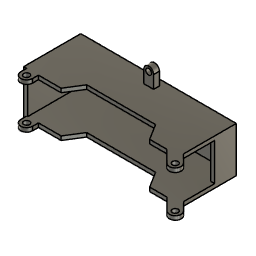
電池ボックス v6 (Autodesk Fusion 360 design; units mm, degrees)
Autodesk Fusion 360 part; units mm, degrees
sketch "スケッチ1" plane through (0, 0, 0) normal (1, 0, 0) x (0, 1, 0)
  line L0 (0, 0) -> (31, 0)
  line L1 (31, 0) -> (31, 25)
  line L2 (31, 25) -> (0, 25)
  line L3 (0, 25) -> (0, 0)
  line L4 (0, 0) -> (0, 12.5)
  line L5 (0, 12.5) -> (0, 2)
  line L6 (0, 12.5) -> (0, 23)
  line L7 (15.5, 0) -> (0, 0)
  line L8 (15.5, 2) -> (2, 2)
  line L9 (15.5, 2) -> (29, 2)
  line L10 (2, 2) -> (2, 23)
  line L11 (29, 2) -> (29, 23)
  line L12 (2, 23) -> (29, 23)
  dimension "d1" = 31
  dimension "d2" = 12.5
  dimension "d3" = 10.5
  dimension "d4" = 10.5
  dimension "d5" = 2
  dimension "d6" = 13.5
  dimension "d7" = 13.5
  dimension "d8" = 21
  dimension "d9" = 21
  constraint horizontal L0
  constraint vertical L1
  constraint horizontal L2
  constraint vertical L3
  constraint coincident L0.start L3.end
  constraint perpendicular L0 L4
  constraint parallel L3 L5
  constraint parallel L3 L6
  constraint midpoint L0 L7.start
  constraint perpendicular L1 L9
  constraint perpendicular L8 L10
  constraint perpendicular L9 L11
  measures "d1" distance of L0.start L0.end
  measures "d2" distance of L0.start L4.end
  measures "d3" distance of L4.end L5.end
  measures "d4" distance of L4.end L6.end
  measures "d5" distance of L7.start L8.start
  measures "d6" distance of L8.start L8.end
  measures "d7" distance of L8.start L9.end
  measures "d8" distance of L8.end L10.end
  measures "d9" distance of L9.end L11.end
extrude "押し出し1" add sketch "スケッチ1" along normal blind 75 makes body 1
sketch "スケッチ2" plane through (0, 31, 0) normal (0, 1, 0) x (-1, 0, 0)
sketch "スケッチ3" plane through (0, 0, 0) normal (1, 0, 0) x (0, 1, 0)
sketch "スケッチ4" plane through (0, 0, 0) normal (0, 1, 0) x (1, 0, 0)
sketch "スケッチ5" plane through (0, 0, 0) normal (1, 0, 0) x (0, 1, 0)
  line L0 (0, 0) -> (2, 0)
  line L1 (2, 0) -> (2, 25)
  line L2 (2, 25) -> (0, 25)
  line L3 (0, 25) -> (0, 0)
  constraint horizontal L0
  constraint vertical L1
  constraint horizontal L2
  constraint vertical L3
  constraint coincident L0.start L3.end
extrude "押し出し2" cut sketch "スケッチ5" along normal blind 75 bodies 1
sketch "スケッチ6" plane through (0, 0, 0) normal (0, 0, 1) x (1, 0, 0)
  circle A0 centre (77, 0) radius 1
  arc A1 (75.5858, -1.4142) -> (78.3586, 1.4677) centre (77, 0) ccw
  line L0 (78.3586, 1.4677) -> (75, 4)
  line L1 (75, 4) -> (75, 2)
  line L2 (75, 2) -> (73, 2)
  line L3 (73, 2) -> (75.5858, -1.4142)
  dimension "d17" = 2
  constraint coincident A0.centre A1.centre
  constraint vertical L1
  constraint perpendicular L1 L2
  measures "d17" radius of A1
extrude "押し出し3" add sketch "スケッチ6" along normal blind 2 bodies 1
sketch "スケッチ7" plane through (0, 0, 25) normal (0, 0, 1) x (-1, 0, 0)
  line L0 (0, -2) -> (-75, -2)
  line L1 (-75, -2) -> (-75, -31)
  line L2 (-75, -31) -> (0, -31)
  line L3 (0, -31) -> (0, -2)
  circle A0 centre (-77, 0) radius 1
  arc A1 (-75.5967, 1.425) -> (-78.4142, -1.4142) centre (-77, 0) ccw
  line L4 (-75.5967, 1.425) -> (-73, -2)
  line L5 (-75, -2) -> (-75, -4)
  line L6 (-78.4142, -1.4142) -> (-75, -4)
  line L7 (-75, -2) -> (-73, -2)
  dimension "d20" = 2
  constraint coincident A0.centre A1.centre
  constraint coincident L0 L4.end
  constraint coincident L0.end L1.start
  constraint coincident L1 L5.end
  constraint perpendicular L0 L5
  measures "d20" radius of A1
extrude "押し出し4" add sketch "スケッチ7" against normal blind 2 contours L0 L1 A1 L4 L5 L6 L7 bodies 1
sketch "スケッチ8" plane through (0, 0, 0) normal (0, 0, 1) x (1, 0, 0)
sketch "スケッチ9" plane through (0, 0, 0) normal (1, 0, 0) x (0, 1, 0)
sketch "スケッチ10" plane through (0, 0, 0) normal (0, 1, 0) x (1, 0, 0)
sketch "スケッチ11" plane through (0, 0, 0) normal (1, 0, 0) x (0, 1, 0)
  line L0 (31, 25) -> (9, 25)
  line L1 (9, 25) -> (9, 0)
  line L2 (9, 0) -> (31, 0)
  line L3 (31, 0) -> (31, 25)
  constraint horizontal L0
  constraint vertical L1
  constraint horizontal L2
  constraint vertical L3
extrude "押し出し5" add sketch "スケッチ11" against normal blind 2 bodies 1
sketch "スケッチ12" plane through (0, 0, 0) normal (1, 0, 0) x (0, 1, 0)
  line L0 (29, 23) -> (17, 23)
  line L1 (2, 23) -> (17, 23)
  line L2 (17, 23) -> (17, 2)
  line L3 (17, 2) -> (2, 2)
  line L4 (2, 2) -> (2, 23)
  constraint horizontal L0
  constraint horizontal L1
  constraint vertical L2
  constraint horizontal L3
  constraint vertical L4
extrude "押し出し6" add sketch "スケッチ12" along normal blind 75 bodies 1
sketch "スケッチ13" plane through (0, 0, 0) normal (1, 0, 0) x (0, 1, 0)
  line L0 (2, 23) -> (17, 23)
  line L1 (17, 23) -> (17, 2)
  line L2 (17, 2) -> (2, 2)
  line L3 (2, 2) -> (2, 23)
  constraint horizontal L0
  constraint vertical L1
  constraint horizontal L2
  constraint vertical L3
extrude "押し出し7" cut sketch "スケッチ13" along normal blind 73 bodies 1
sketch "スケッチ14" plane through (0, 0, 25) normal (0, 0, 1) x (-1, 0, 0)
  circle A0 centre (-77, 0) radius 1
  line L0 (0, -2) -> (-73, -2)
  line L1 (-73, -2) -> (-75.5967, 1.425)
  arc A1 (-75.5967, 1.425) -> (-78.4142, -1.4142) centre (-77, 0) ccw
  line L2 (-78.4142, -1.4142) -> (-75, -4)
  line L3 (-75, -4) -> (-75, -31)
  line L4 (-75, -31) -> (2, -31)
  line L5 (2, -31) -> (2, -9)
  line L6 (2, -9) -> (0, -9)
  line L7 (0, -9) -> (0, -2)
  line L8 (0, -2) -> (-3, -2)
  line L9 (0, -2) -> (0, 1.5)
  line L10 (-3, -2) -> (-3, 1.5)
  circle A2 centre (-1.5, 1.5) radius 1
  arc A3 (0, 1.5) -> (-3, 1.5) centre (-1.5, 1.5) ccw
  constraint coincident L0.start L7.end
  constraint coincident L0 L8.end
  constraint perpendicular L7 L8
  constraint perpendicular L0 L9
  constraint perpendicular L8 L10
  constraint coincident A2.centre A3.centre
extrude "押し出し8" add sketch "スケッチ14" against normal blind 25 contours L0 L8 L9 L10 A3 bodies 1
sketch "スケッチ15" plane through (0, 0, 25) normal (0, 0, 1) x (-1, 0, 0)
  circle A0 centre (-1.5, 1.5) radius 1
  circle A1 centre (-77, 0) radius 1
  line L0 (-3, -2) -> (-73, -2)
  line L1 (-73, -2) -> (-75.5967, 1.425)
  arc A2 (-75.5967, 1.425) -> (-78.4142, -1.4142) centre (-77, 0) ccw
  line L2 (-78.4142, -1.4142) -> (-75, -4)
  line L3 (-75, -4) -> (-75, -31)
  line L4 (-75, -31) -> (2, -31)
  line L5 (2, -31) -> (2, -9)
  line L6 (2, -9) -> (0, -9)
  line L7 (0, -9) -> (0, 1.5)
  arc A3 (0, 1.5) -> (-3, 1.5) centre (-1.5, 1.5) ccw
  line L8 (-3, 1.5) -> (-3, -2)
  line L9 (-3, 1.5) -> (-3, -2)
  line L10 (0, -2) -> (-3, -2)
  line L11 (0, -2) -> (0, 1.5)
  arc A4 (0, 1.5) -> (-3, 1.5) centre (-1.5, 1.5) ccw
  circle A5 centre (-1.5, 1.5) radius 1
  constraint coincident A3.end L8.start
  constraint coincident L0.start L8.end
  constraint coincident L7 L10.start
  constraint perpendicular L8 L10
  constraint coincident L7.end A3.start
  constraint coincident A0.centre A3.centre
  constraint concentric A4 A5
extrude "押し出し9" cut sketch "スケッチ15" against normal blind 23 contours L7 A3 L8 L9 L10 L11 A4 bodies 1
sketch "スケッチ16" plane through (0, 0, 25) normal (0, 0, 1) x (-1, 0, 0)
  line L0 (0, -2) -> (-73, -2)
  line L1 (-73, -2) -> (-75.5967, 1.425)
  arc A0 (-75.5967, 1.425) -> (-78.4142, -1.4142) centre (-77, 0) ccw
  line L2 (-78.4142, -1.4142) -> (-75, -4)
  line L3 (-75, -4) -> (-75, -31)
  line L4 (-75, -31) -> (2, -31)
  line L5 (2, -31) -> (2, -9)
  line L6 (2, -9) -> (0, -9)
  line L7 (0, -9) -> (0, -2)
  circle A1 centre (-77, 0) radius 1
  line L8 (-3, 1.5) -> (-3, -2)
  line L9 (-3, -2) -> (0, -2)
  line L10 (0, 1.5) -> (0, -2)
  arc A2 (0, 1.5) -> (-3, 1.5) centre (-1.5, 1.5) ccw
  circle A3 centre (-1.5, 1.5) radius 1
  constraint coincident L0 L8.end
  constraint perpendicular L0 L8
  constraint coincident L0.start L7.end
  constraint perpendicular L0 L10
  constraint concentric A2 A3
extrude "押し出し10" add sketch "スケッチ16" against normal blind 2 contours L0 L8 L9 L10 A2 bodies 1
sketch "スケッチ17" plane through (0, 0, 25) normal (0, 0, 1) x (-1, 0, 0)
  circle A0 centre (-1.5, 1.5) radius 1
  line L0 (-3, -2) -> (-73, -2)
  line L1 (-73, -2) -> (-75.5967, 1.425)
  arc A1 (-75.5967, 1.425) -> (-78.4142, -1.4142) centre (-77, 0) ccw
  line L2 (-78.4142, -1.4142) -> (-75, -4)
  line L3 (-75, -4) -> (-75, -31)
  line L4 (-75, -31) -> (2, -31)
  line L5 (2, -31) -> (2, -9)
  line L6 (2, -9) -> (0, -9)
  line L7 (0, -9) -> (0, 1.5)
  arc A2 (0, 1.5) -> (-3, 1.5) centre (-1.5, 1.5) ccw
  line L8 (-3, 1.5) -> (-3, -2)
  circle A3 centre (-77, 0) radius 1
  circle A4 centre (4, 1) radius 0.95
  dimension "d35" = 1.9
  measures "d35" diameter of A4
sketch "スケッチ18" plane through (0, 0, 0) normal (0, 0, 1) x (1, 0, 0)
  circle A0 centre (-6.5, -1) radius 0.95
  dimension "d38" = 1.9
  measures "d38" diameter of A0
sketch "スケッチ19" plane through (0, 31, 0) normal (0, 1, 0) x (-1, 0, 0)
sketch "スケッチ20" plane through (0, 0, 0) normal (0, 0, 1) x (1, 0, 0)
  line L0 (15, 2) -> (20, 10)
  line L1 (20, 10) -> (55, 10)
  line L2 (55, 10) -> (60, 2)
  line L3 (15, 2) -> (60, 2)
  constraint horizontal L1
  constraint horizontal L3
extrude "押し出し13" cut sketch "スケッチ20" along normal blind 2 bodies 1
sketch "スケッチ21" plane through (0, 0, 25) normal (0, 0, 1) x (-1, 0, 0)
  circle A0 centre (-1.5, 1.5) radius 1
  line L0 (-3, -2) -> (-73, -2)
  line L1 (-73, -2) -> (-75.5967, 1.425)
  arc A1 (-75.5967, 1.425) -> (-78.4142, -1.4142) centre (-77, 0) ccw
  line L2 (-78.4142, -1.4142) -> (-75, -4)
  line L3 (-75, -4) -> (-75, -31)
  line L4 (-75, -31) -> (2, -31)
  line L5 (2, -31) -> (2, -9)
  line L6 (2, -9) -> (0, -9)
  line L7 (0, -9) -> (0, 1.5)
  arc A2 (0, 1.5) -> (-3, 1.5) centre (-1.5, 1.5) ccw
  line L8 (-3, 1.5) -> (-3, -2)
  circle A3 centre (-77, 0) radius 1
  line L9 (-15, -2) -> (-20, -10)
  line L10 (-60, -2) -> (-55, -10)
  line L11 (-55, -10) -> (-20, -10)
  constraint coincident L0 L9.start
  constraint coincident L0 L10.start
  constraint parallel L0 L11
extrude "押し出し14" cut sketch "スケッチ21" against normal blind 2 contours L0 L9 L10 L11 bodies 1
sketch "スケッチ22" plane through (0, 0, 0) normal (0, 0, 1) x (1, 0, 0)
sketch "スケッチ23" plane through (0, 31, 0) normal (0, 1, 0) x (-1, 0, 0)
sketch "スケッチ24" plane through (0, 0, 0) normal (0, 0, 1) x (1, 0, 0)
sketch "スケッチ25" plane through (0, 0, 0) normal (0, 1, 0) x (1, 0, 0)
  line L0 (75, 0) -> (36.5, 0)
  line L1 (36.5, 0) -> (36.5, -25)
  line L2 (36.5, 0) -> (34, 0)
  line L3 (36.5, 0) -> (39, 0)
  line L4 (39, 0) -> (34, 0)
  line L5 (34, 0) -> (34, 8)
  line L6 (34, 8) -> (39, 8)
  line L7 (39, 8) -> (39, 0)
  line L8 (34, 8) -> (34, 5.5)
  line L9 (34, 5.5) -> (36.5, 5.5)
  circle A0 centre (36.5, 5.5) radius 1.5
  arc A1 (39, 5.4984) -> (34, 5.5) centre (36.5, 5.5) ccw
  dimension "d46" = 38.5
  dimension "d47" = 2.5
  dimension "d48" = 2.5
  dimension "d49" = 2.5
  dimension "d50" = 2.5
  dimension "d51" = 3
  constraint horizontal L0
  constraint perpendicular L0 L1
  constraint perpendicular L1 L2
  constraint perpendicular L1 L3
  constraint horizontal L4
  constraint vertical L5
  constraint horizontal L6
  constraint vertical L7
  constraint perpendicular L6 L8
  constraint perpendicular L7 L9
  constraint coincident L9.end A0.centre
  constraint coincident L7 A1.start
  measures "d46" distance of L0.start L0.end
  measures "d47" distance of L0.end L2.end
  measures "d48" distance of L0.end L3.end
  measures "d49" distance of L5.end L8.end
  measures "d50" distance of L8.end L9.end
  measures "d51" diameter of A0
extrude "押し出し15" add sketch "スケッチ25" along normal blind 15 contours L0 L2 L3 L4 L5 L7 A1 bodies 1
extrude "押し出し16" cut 1 faces at (36.4626, 0, -1.3347) along direction (0, 1, 0) blind 13 on bodies 1 bodies 1
sketch "スケッチ26" plane through (0, 0, 0) normal (0, 1, 0) x (1, 0, 0)
  line L0 (-2, -25) -> (36.5, -25)
  line L1 (36.5, -25) -> (36.5, -30.5)
  circle A0 centre (36.5, -30.5) radius 1.5
  arc A1 (34, -30.5) -> (39, -30.5) centre (36.5, -30.5) ccw
  line L2 (34, -30.5) -> (34, -25)
  line L3 (39.2947, -30.5) -> (39.2947, -25)
  line L4 (39.2947, -25) -> (34, -25)
  line L5 (39, -30.5) -> (39, -25)
  dimension "d56" = 38.5
  dimension "d57" = 5.5
  dimension "d58" = 3
  dimension "d59" = 2.5
  constraint horizontal L0
  constraint perpendicular L0 L1
  constraint coincident L1.end A0.centre
  constraint coincident L0 L2.end
  constraint tangent A1 L2
  constraint perpendicular L0 L2
  constraint parallel L2 L3
  constraint perpendicular L2 L4
  constraint coincident L4 L5.end
  constraint tangent A1 L5
  constraint perpendicular L4 L5
  measures "d56" distance of L0.start L0.end
  measures "d57" distance of L0.end L1.end
  measures "d58" diameter of A0
  measures "d59" radius of A1
extrude "押し出し17" add sketch "スケッチ26" along normal blind 15 bodies 1
extrude "押し出し18" cut 1 faces at (36.5374, 0, 26.3347) along direction (0, 1, 0) blind 20 on bodies 1 bodies 1
sketch "スケッチ27" plane through (0, 0, 0) normal (0, 1, 0) x (1, 0, 0)
sketch "スケッチ28" plane through (0, 0, 0) normal (0, 1, 0) x (1, 0, 0)
  line L0 (-2, -2) -> (-2, -21)
  line L1 (-2, -21) -> (75, -21)
  line L2 (75, -23) -> (75, -21)
  line L3 (75, -23) -> (-2, -23)
  line L4 (-2, -23) -> (-2, -21)
  constraint vertical L0
  constraint perpendicular L0 L1
  constraint perpendicular L1 L2
  constraint perpendicular L2 L3
  constraint perpendicular L1 L4
extrude "押し出し19" cut sketch "スケッチ28" along normal blind 70 bodies 1 makes body 2 at (38, 25.6667, 0)
move_body "移動4" bodies 1 to x (1, 0, 0) y (0, 1, 0) z (0, 0, 1) at (0, 0, -2)
sketch "スケッチ29" plane through (0, 0, 0) normal (0, 1, 0) x (1, 0, 0)
sketch "スケッチ30" plane through (0, 13, 0) normal (0, -1, 0) x (1, 0, 0)
extrude "押し出し20" cut 1 faces at (36.4626, 15, -1.3347) along direction (0, -1, 0) blind 40 on bodies 2 bodies 2
sketch "スケッチ31" plane through (0, 0, 0) normal (0, 1, 0) x (1, 0, 0)
  line L0 (39, 0) -> (39, 4)
  line L1 (39, 0) -> (34, 0)
  line L2 (34, 0) -> (34, 4)
  circle A0 centre (36.5, 6.5) radius 1.5
  arc A1 (39, 6.5) -> (34, 6.5) centre (36.5, 6.5) ccw
  line L3 (34, 6.5) -> (34, 4)
  line L4 (39, 6.5) -> (39, 4)
  constraint vertical L0
  constraint perpendicular L0 L1
  constraint perpendicular L1 L2
  constraint coincident A0.centre A1.centre
  constraint parallel L2 L3
extrude "押し出し21" add sketch "スケッチ31" along normal blind 14 bodies 2
extrude "押し出し22" cut 1 faces at (36.5374, 0, -1.6681) along direction (0, 1, 0) blind 12 on bodies 2 bodies 2
sketch "スケッチ32" plane through (0, 29, 0) normal (0, -1, 0) x (1, 0, 0)
  line L0 (75, 21) -> (0, 21)
  line L1 (0, 21) -> (0, 2)
  line L2 (0, 2) -> (75, 2)
  line L3 (75, 2) -> (75, 21)
  line L4 (39, 23) -> (39, 27)
  line L5 (34, 23) -> (34, 27)
  line L6 (34, 23) -> (39, 23)
  circle A0 centre (36.5, 29.5) radius 1.5
  arc A1 (39, 29.5) -> (34, 29.5) centre (36.5, 29.5) ccw
  line L7 (39, 29.5) -> (39, 27)
  line L8 (34, 29.5) -> (34, 27)
  dimension "d78" = 3
  constraint perpendicular L0 L4
  constraint vertical L5
  constraint perpendicular L4 L6
  constraint coincident A0.centre A1.centre
  constraint parallel L4 L7
  constraint parallel L5 L8
  measures "d78" diameter of A0
extrude "押し出し23" add sketch "スケッチ32" along normal blind 17 contours L4 L5 L6 A1 L7 L8 bodies 1
extrude "押し出し24" cut 1 faces at (36.5374, 29, 24.6681) along direction (0, -1, 0) blind 15 on bodies 1 bodies 1
sketch "スケッチ33" plane through (0, 0, 0) normal (0, 1, 0) x (1, 0, 0)
sketch "スケッチ34" plane through (0, 0, 0) normal (0, 1, 0) x (1, 0, 0)
sketch "スケッチ35" plane through (0, 0, 0) normal (0, 1, 0) x (1, 0, 0)
sketch "スケッチ36" plane through (0, 0, 23) normal (0, 0, 1) x (-1, 0, 0)
sketch "スケッチ37" plane through (0, 0, 0) normal (1, 0, 0) x (0, 1, 0)
sketch "スケッチ38" plane through (0, 0, 2) normal (0, 0, 1) x (-1, 0, 0)
sketch "スケッチ39" plane through (0, 0, 0) normal (0, 1, 0) x (1, 0, 0)
move_body "移動5" bodies 2 1 to x (1, 0, 0) y (0, 1, 0) z (0, 0, 1) at (2, 0, 0)
sketch "スケッチ40" plane through (0, 0, 0) normal (1, 0, 0) x (0, 1, 0)
  line L0 (9, 23) -> (31, 23)
  line L1 (31, 23) -> (31, 0)
  line L2 (31, 0) -> (9, 0)
  line L3 (9, 0) -> (9, 23)
  constraint horizontal L0
  constraint vertical L1
  constraint horizontal L2
  constraint vertical L3
extrude "押し出し25" cut sketch "スケッチ40" along normal blind 2 bodies 1 2
sketch "スケッチ41" plane through (0, 0, 0) normal (0, 0, 1) x (1, 0, 0)
  line L0 (5, 2) -> (0.471, 2)
  line L1 (0.471, 2) -> (0.471, -4.3481)
  line L2 (0.471, -4.3481) -> (5, -4.3481)
  line L3 (5, -4.3481) -> (5, 2)
  constraint horizontal L0
  constraint vertical L1
  constraint horizontal L2
  constraint vertical L3
extrude "押し出し26" cut sketch "スケッチ41" along normal blind 30 bodies 1 2
extrude "押し出し27" add 1 faces at (2, 19, 22.3333) along direction (-1, 0, 0) blind 2 on bodies 1 bodies 1 2
extrude "押し出し28" add 1 faces at (2, 16.6667, 0.6667) along direction (-1, 0, 0) blind 2 on bodies 1 bodies 1
sketch "スケッチ42" plane through (0, 0, 0) normal (1, 0, 0) x (0, 1, 0)
  line L0 (31, 23) -> (2, 23)
  line L1 (2, 23) -> (2, 0)
  line L2 (2, 0) -> (31, 0)
  line L3 (31, 0) -> (31, 23)
  constraint horizontal L0
  constraint vertical L1
  constraint horizontal L2
  constraint vertical L3
extrude "押し出し29" add sketch "スケッチ42" against normal blind 2 bodies 1
sketch "スケッチ43" plane through (0, 2, 0) normal (0, -1, 0) x (1, 0, 0)
sketch "スケッチ44" plane through (0, 0, 0) normal (1, 0, 0) x (0, 1, 0)
  line L0 (2, 21) -> (14, 21)
  line L1 (14, 21) -> (14, 2)
  line L2 (14, 2) -> (2, 2)
  line L3 (2, 2) -> (2, 21)
  constraint horizontal L0
  constraint vertical L1
  constraint horizontal L2
  constraint vertical L3
extrude "押し出し30" cut sketch "スケッチ44" against normal blind 2 bodies 1
sketch "スケッチ45" plane through (0, 0, 0) normal (0, 0, 1) x (1, 0, 0)
  line L0 (0, 15) -> (-2, 15)
  line L1 (-2, 15) -> (-2, 2)
  line L2 (-2, 2) -> (0, 2)
  line L3 (0, 2) -> (0, 15)
  constraint horizontal L0
  constraint vertical L1
  constraint horizontal L2
  constraint vertical L3
extrude "押し出し31" cut sketch "スケッチ45" along normal blind 100 bodies 1
sketch "スケッチ46" plane through (0, 2, 0) normal (0, -1, 0) x (1, 0, 0)
sketch "スケッチ47" plane through (0, 0, 0) normal (0, 0, 1) x (1, 0, 0)
  line L0 (0, 2) -> (5, 2)
  line L1 (5, 2) -> (5, -2)
  line L2 (0, 2) -> (0, -2)
  circle A0 centre (2.5, -1) radius 1.5
  arc A1 (0, -1) -> (5, -1) centre (2.5, -1) ccw
  constraint horizontal L0
  constraint perpendicular L0 L1
  constraint perpendicular L0 L2
  constraint coincident L1 A1.end
  constraint coincident L2 A1.start
  constraint coincident A0.centre A1.centre
extrude "押し出し32" add sketch "スケッチ47" along normal blind 23 bodies 1
sketch "スケッチ48" plane through (0, 0, 0) normal (0, 1, 0) x (1, 0, 0)
  line L0 (0, -21) -> (5, -21)
  line L1 (5, -21) -> (5, -2)
  line L2 (5, -2) -> (0, -2)
  line L3 (0, -2) -> (0, -21)
  constraint horizontal L0
  constraint vertical L1
  constraint horizontal L2
  constraint vertical L3
extrude "押し出し33" cut sketch "スケッチ48" against normal blind 10 bodies 1
sketch "スケッチ49" plane through (0, 0, 0) normal (0, 1, 0) x (1, 0, 0)
  line L0 (0, -2) -> (5, -2)
  line L1 (5, -2) -> (5, -21)
  line L2 (5, -21) -> (0, -21)
  line L3 (0, -21) -> (0, -2)
  constraint horizontal L0
  constraint vertical L1
  constraint horizontal L2
  constraint vertical L3
extrude "押し出し34" cut sketch "スケッチ49" along normal blind 9 bodies 1
sketch "スケッチ50" plane through (0, 0, 0) normal (0, 0, 1) x (1, 0, 0)
  line L0 (77, 31) -> (49, 31)
  line L1 (49, 31) -> (49, 2)
  line L2 (49, 2) -> (77, 2)
  line L3 (77, 2) -> (77, 31)
  line L4 (77, 4) -> (77, 2)
  line L5 (75, 2) -> (77, 2)
  line L6 (77, 4) -> (81.5, 4)
  line L7 (81.5, 4) -> (81.5, -2.5)
  line L8 (81.5, -2.5) -> (75, -2.5)
  line L9 (75, -2.5) -> (75, 2)
  constraint horizontal L0
  constraint vertical L1
  constraint horizontal L2
  constraint vertical L3
  constraint coincident L3 L4.start
  constraint coincident L2 L5.start
  constraint perpendicular L3 L6
  constraint perpendicular L6 L7
  constraint perpendicular L7 L8
extrude "押し出し35" cut sketch "スケッチ50" along normal blind 30 contours L2 L3 L4 L5 L6 L7 L8 L9 bodies 1
sketch "スケッチ51" plane through (0, 0, 0) normal (0, 0, 1) x (1, 0, 0)
  circle A0 centre (79, 0) radius 1.5
  arc A1 (77.2322, -1.7678) -> (80.7678, 1.7678) centre (79, 0) ccw
  line L0 (79, 0) -> (77.2322, -1.7678) construction
  line L1 (79, 0) -> (80.7678, 1.7678) construction
  line L2 (77, 2) -> (77, 7.5)
  line L3 (77, 2) -> (72.5, 2)
  line L4 (80.7678, 1.7678) -> (77, 5.5355)
  line L5 (77.2322, -1.7678) -> (73.4645, 2)
  line L6 (77, 2) -> (75, 2)
  line L7 (75, 0.4645) -> (75, 2)
  dimension "d105" = 2.5
  dimension "d106" = 180
  constraint coincident A0.centre A1.centre
  constraint vertical L2
  constraint perpendicular L2 L3
  constraint coincident L2 L4.end
  constraint tangent A1 L4
  constraint coincident L3 L5.end
  constraint tangent A1 L5
  constraint coincident L3 L6.end
  constraint coincident L5 L7.start
  constraint perpendicular L6 L7
  measures "d105" radius of A1
  measures "d106" angle of L0 L1
extrude "押し出し36" add sketch "スケッチ51" along normal blind 23 contours A1 L2 L3 L4 L5 L6 L7 bodies 1
sketch "スケッチ52" plane through (0, 0, 0) normal (0, 0, 1) x (1, 0, 0)
sketch "スケッチ53" plane through (0, 0, 0) normal (0, 1, 0) x (1, 0, 0)
  line L0 (75, -2) -> (82, -2)
  line L1 (82, -2) -> (82, -21)
  line L2 (82, -21) -> (75, -21)
  line L3 (75, -21) -> (75, -2)
  constraint horizontal L0
  constraint vertical L1
  constraint horizontal L2
  constraint vertical L3
extrude "押し出し37" cut sketch "スケッチ53" against normal blind 5 bodies 1
sketch "スケッチ54" plane through (0, 0, 0) normal (0, 0, 1) x (1, 0, 0)
sketch "スケッチ55" plane through (0, 0, 0) normal (0, 1, 0) x (1, 0, 0)
  line L0 (75, -2) -> (82, -2)
  line L1 (82, -2) -> (82, -21)
  line L2 (82, -21) -> (75, -21)
  line L3 (75, -21) -> (75, -2)
  constraint horizontal L0
  constraint vertical L1
  constraint horizontal L2
  constraint vertical L3
extrude "押し出し38" cut sketch "スケッチ55" along normal blind 2 bodies 1
sketch "スケッチ56" plane through (0, 0, 0) normal (0, 1, 0) x (1, 0, 0)
  line L0 (75, -21) -> (77, -21)
  line L1 (77, -21) -> (84, -21)
  line L2 (84, -21) -> (84, -2)
  line L3 (84, -2) -> (77, -2)
  line L4 (77, -2) -> (77, -21)
  constraint horizontal L0
  constraint horizontal L1
  constraint vertical L2
  constraint horizontal L3
  constraint vertical L4
extrude "押し出し39" cut sketch "スケッチ56" along normal blind 55555 bodies 1
sketch "スケッチ57" plane through (0, 0, 0) normal (0, 0, 1) x (1, 0, 0)
sketch "スケッチ58" plane through (0, 0, 0) normal (0, 0, 1) x (1, 0, 0)
sketch "スケッチ59" plane through (0, 0, 0) normal (0, 1, 0) x (1, 0, 0)
sketch "スケッチ60" plane through (0, 0, 0) normal (0, 0, 1) x (1, 0, 0)
sketch "スケッチ61" plane through (0, 0, 0) normal (0, 0, 1) x (1, 0, 0)
sketch "スケッチ62" plane through (0, 0, 0) normal (0, 0, 1) x (1, 0, 0)
sketch "スケッチ63" plane through (0, 0, 0) normal (0, 0, 1) x (1, 0, 0)
  line L0 (77, 5.55) -> (77, 2)
  line L1 (77, 2) -> (74.5, 2)
  line L2 (74.5, 2) -> (74.5, -4)
  line L3 (74.5, -4) -> (83, -4)
  line L4 (83, -4) -> (83, 6.3371)
  line L5 (83, 6.3371) -> (77, 5.55)
  constraint vertical L0
  constraint perpendicular L0 L1
  constraint perpendicular L1 L2
  constraint perpendicular L0 L3
  constraint perpendicular L3 L4
extrude "押し出し40" cut sketch "スケッチ63" along normal blind 90 bodies 1
sketch "スケッチ64" plane through (0, 0, 0) normal (0, 0, 1) x (1, 0, 0)
  circle A0 centre (79, -2) radius 1.5
  arc A1 (77.2335, -3.769) -> (80.7665, -0.231) centre (79, -2) ccw
  line L0 (79, -2) -> (77.2335, -3.769) construction
  line L1 (79, -2) -> (80.7665, -0.231) construction
  line L2 (77.2335, -3.769) -> (71, 2)
  line L3 (71, 2) -> (77, 2)
  line L4 (77, 2) -> (77, 6.6647)
  line L5 (80.7665, -0.231) -> (77, 3.5301)
  dimension "d117" = 3
  dimension "d118" = 2.5
  dimension "d119" = 180
  constraint perpendicular L3 L4
  constraint coincident L4 L5.end
  constraint tangent A1 L5
  measures "d117" diameter of A0
  measures "d118" radius of A1
  measures "d119" angle of L0 L1
extrude "押し出し41" add sketch "スケッチ64" along normal blind 23 bodies 1
sketch "スケッチ65" plane through (0, 0, 0) normal (0, 0, 1) x (1, 0, 0)
move_body "移動6" bodies 1 to x (1, 0, 0) y (0, 1, 0) z (0, 0, 1) at (0, -2, 0)
sketch "スケッチ66" plane through (0, 0, 0) normal (0, 1, 0) x (1, 0, 0)
  line L0 (69, -2) -> (92, -2)
  line L1 (92, -2) -> (92, -21)
  line L2 (92, -21) -> (69, -21)
  line L3 (69, -21) -> (69, -2)
  constraint horizontal L0
  constraint vertical L1
  constraint horizontal L2
  constraint vertical L3
extrude "押し出し42" cut sketch "スケッチ66" against normal blind 90 bodies 1
sketch "スケッチ67" plane through (0, 0, 0) normal (1, 0, 0) x (0, 1, 0)
sketch "スケッチ68" plane through (0, 0, 0) normal (0, 1, 0) x (1, 0, 0)
  line L0 (77, -2) -> (88, -2)
  line L1 (88, -2) -> (88, -21)
  line L2 (88, -21) -> (77, -21)
  line L3 (77, -21) -> (77, -2)
  constraint horizontal L0
  constraint vertical L1
  constraint horizontal L2
  constraint vertical L3
extrude "押し出し43" cut sketch "スケッチ68" along normal blind 10 bodies 1
extrude "押し出し44" add 1 faces at (38.5374, 12, -1.6681) along direction (0, 1, 0) blind 14 on bodies 1 bodies 1
extrude "押し出し45" add 1 faces at (38.5374, 12, 24.6681) along direction (0, 1, 0) blind 14 on bodies 1 bodies 1
extrude "押し出し46" cut 1 faces at (38.5374, 10, 24.6681) along direction (0, 1, 0) blind 14 on bodies 1 bodies 1
extrude "押し出し47" cut 1 faces at (38.5374, 10, -1.6681) along direction (0, 1, 0) blind 14 on bodies 1 bodies 1
sketch "スケッチ69" plane through (0, 0, 0) normal (1, 0, 0) x (0, 1, 0)
  line L0 (13, 23) -> (2, 23)
  line L1 (2, 23) -> (2, 0)
  line L2 (2, 0) -> (13, 0)
  line L3 (13, 0) -> (13, 23)
  constraint horizontal L0
  constraint vertical L1
  constraint horizontal L2
  constraint vertical L3
extrude "押し出し48" add sketch "スケッチ69" against normal blind 2 bodies 1
sketch "スケッチ70" plane through (0, 0, 0) normal (0, 0, 1) x (1, 0, 0)
extrude "押し出し49" add 1 faces at (38.5374, 24, 24.6681) along direction (0, -1, 0) blind 1 on bodies 1 bodies 1
extrude "押し出し50" add 1 faces at (38.5374, 24, -1.6681) along direction (0, -1, 0) blind 1 on bodies 1 bodies 1
extrude "押し出し51" cut 1 faces at (38.5374, 26, -1.6681) along direction (0, -1, 0) blind 1 on bodies 1 bodies 1
extrude "押し出し52" cut 1 faces at (38.5374, 26, 24.6681) along direction (0, -1, 0) blind 1 on bodies 1 bodies 1
sketch "スケッチ71" plane through (0, 0, 0) normal (0, 1, 0) x (1, 0, 0)
sketch "スケッチ72" plane through (0, 0, 0) normal (0, 0, 1) x (1, 0, 0)
  line L0 (70.7, 0) -> (77, 0)
  line L1 (77, 0) -> (77, 2)
  line L2 (77, 2) -> (84, -5)
  line L3 (84, -5) -> (78.3332, -8.0341)
  line L4 (78.3332, -8.0341) -> (70.7, 0)
  constraint horizontal L0
  constraint perpendicular L0 L1
extrude "押し出し53" cut sketch "スケッチ72" along normal blind 90 bodies 1
sketch "スケッチ73" plane through (0, 0, 0) normal (0, 0, 1) x (1, 0, 0)
  line L0 (77, 0) -> (77, -2)
  line L1 (77, -2) -> (79, -4)
  circle A0 centre (79, -4) radius 1.5
  arc A1 (76.8723, -6.1149) -> (81.1277, -1.8851) centre (79, -4) ccw
  line L2 (79, -4) -> (76.8723, -6.1149) construction
  line L3 (79, -4) -> (81.1277, -1.8851) construction
  line L4 (77, 0) -> (71, 0)
  line L5 (77, 0) -> (77, 5.3272)
  line L6 (76.8723, -6.1149) -> (70.7943, 0)
  line L7 (70.7943, 0) -> (71, 0)
  line L8 (81.1277, -1.8851) -> (77, 2.2677)
  dimension "d146" = 3
  dimension "d147" = 3
  dimension "d148" = 180
  constraint vertical L0
  constraint coincident L1.end A0.centre
  constraint perpendicular L0 L4
  constraint perpendicular L4 L5
  constraint tangent A1 L6
  constraint parallel L4 L7
  constraint coincident L5 L8.end
  constraint perpendicular L3 L8
  measures "d146" diameter of A0
  measures "d147" radius of A1
  measures "d148" angle of L2 L3
extrude "押し出し54" add sketch "スケッチ73" along normal blind 2 bodies 1
move_body "移動7" bodies 1 to x (1, 0, 0) y (0, 1, 0) z (0, 0, 1) at (0, 0, -23)
sketch "スケッチ74" plane through (0, 0, 0) normal (0, 0, 1) x (1, 0, 0)
  line L0 (77, 0) -> (77, -2)
  line L1 (77, -2) -> (79, -4)
  circle A0 centre (79, -4) radius 1.5
  arc A1 (76.9035, -6.1459) -> (81.0965, -1.8541) centre (79, -4) ccw
  line L2 (79, -4) -> (76.9035, -6.1459) construction
  line L3 (79, -4) -> (81.0965, -1.8541) construction
  line L4 (77, 3) -> (77, 0)
  line L5 (81.0965, -1.8541) -> (77, 2.1481)
  line L6 (76.9035, -6.1459) -> (70.7, 0)
  line L7 (77, 0) -> (70.7, 0)
  dimension "d151" = 3
  dimension "d152" = 3
  dimension "d153" = 180
  constraint vertical L0
  constraint coincident L1.end A0.centre
  constraint parallel L0 L4
  constraint coincident L4 L5.end
  constraint tangent A1 L5
  constraint perpendicular L0 L7
  measures "d151" diameter of A0
  measures "d152" radius of A1
  measures "d153" angle of L2 L3
extrude "押し出し55" add sketch "スケッチ74" against normal blind 2 bodies 1
sketch "スケッチ75" plane through (0, 0, 0) normal (1, 0, 0) x (0, 1, 0)
  line L0 (13, 0) -> (2, 0)
  line L1 (2, 0) -> (2, -23)
  line L2 (2, -23) -> (13, -23)
  line L3 (13, -23) -> (13, 0)
  constraint horizontal L0
  constraint vertical L1
  constraint horizontal L2
  constraint vertical L3
extrude "押し出し56" cut sketch "スケッチ75" against normal blind 2 bodies 1
sketch "スケッチ76" plane through (0, 0, 0) normal (0, 0, 1) x (1, 0, 0)
  circle A0 centre (2.5, -3) radius 1.5
  line L0 (0, 0) -> (6.3566, 0)
  line L1 (6.3566, 0) -> (6.3566, -5.9724)
  line L2 (6.3566, -5.9724) -> (0, -5.9724)
  line L3 (0, -5.9724) -> (0, 0)
  constraint horizontal L0
  constraint vertical L1
  constraint horizontal L2
  constraint vertical L3
  constraint coincident L0.start L3.end
extrude "押し出し57" cut sketch "スケッチ76" against normal blind 60 bodies 1
sketch "スケッチ77" plane through (0, 0, 0) normal (0, 0, 1) x (1, 0, 0)
  line L0 (0, 0) -> (2.5, 0)
  line L1 (2.5, 0) -> (2.5, -3)
  circle A0 centre (2.5, -3) radius 1.5
  arc A1 (-0.5, -3) -> (5.5, -3) centre (2.5, -3) ccw
  line L2 (5.5, -3) -> (5.5, 0)
  line L3 (5.5, 0) -> (-0.5, 0)
  line L4 (-0.5, 0) -> (-0.5, -3)
  dimension "d160" = 2.5
  dimension "d161" = 3
  dimension "d162" = 3
  dimension "d163" = 3
  dimension "d164" = 6
  constraint coincident L0.start origin
  constraint horizontal L0
  constraint perpendicular L0 L1
  constraint coincident L1.end A0.centre
  constraint vertical L2
  constraint perpendicular L2 L3
  constraint tangent A1 L4
  measures "d160" distance of L0.start L0.end
  measures "d161" distance of L0.end L1.end
  measures "d162" radius of A1
  measures "d163" distance of A1.end L2.end
  measures "d164" distance of L2.end L3.end
extrude "押し出し58" add sketch "スケッチ77" against normal blind 23 bodies 1
sketch "スケッチ78" plane through (0, 0, 0) normal (0, 1, 0) x (1, 0, 0)
  line L0 (6, 21) -> (-4, 21)
  line L1 (-4, 21) -> (-4, 2)
  line L2 (-4, 2) -> (6, 2)
  line L3 (6, 2) -> (6, 21)
  constraint horizontal L0
  constraint vertical L1
  constraint horizontal L2
  constraint vertical L3
extrude "押し出し59" cut sketch "スケッチ78" against normal blind 90 bodies 1
sketch "スケッチ79" plane through (0, 0, 0) normal (0, 0, 1) x (1, 0, 0)
  line L0 (0, 13) -> (-2, 13)
  line L1 (-2, 13) -> (-2, 0)
  line L2 (-2, 0) -> (0, 0)
  line L3 (0, 0) -> (0, 13)
  constraint horizontal L0
  constraint vertical L1
  constraint horizontal L2
  constraint vertical L3
extrude "押し出し60" add sketch "スケッチ79" against normal blind 23 bodies 1
sketch "スケッチ80" plane through (0, 0, 0) normal (1, 0, 0) x (0, 1, 0)
move_body "移動8" bodies 1 to x (1, 0, 0) y (0, 1, 0) z (0, 0, 1) at (-77, 0, 0)
sketch "スケッチ81" plane through (0, 0, 0) normal (1, 0, 0) x (0, 1, 0)
  line L0 (15, -2) -> (27, -2)
  line L1 (27, -2) -> (27, -21)
  line L2 (27, -21) -> (15, -21)
  line L3 (15, -21) -> (15, -2)
  constraint horizontal L0
  constraint vertical L1
  constraint horizontal L2
  constraint vertical L3
extrude "押し出し61" add sketch "スケッチ81" against normal blind 2 bodies 1
sketch "スケッチ82" plane through (0, 0, 0) normal (1, 0, 0) x (0, 1, 0)
  line L0 (3, -2) -> (15, -2)
  line L1 (15, -2) -> (15, -21)
  line L2 (15, -21) -> (3, -21)
  line L3 (3, -21) -> (3, -2)
  constraint horizontal L0
  constraint vertical L1
  constraint horizontal L2
  constraint vertical L3
extrude "押し出し62" cut sketch "スケッチ82" against normal blind 2 bodies 1
extrude "押し出し63" add 1 faces at (-38.4626, 25, 1.6681) along direction (0, 1, 0) blind 1 on bodies 1 bodies 1
extrude "押し出し64" add 1 faces at (-38.4626, 25, -24.6681) along direction (0, 1, 0) blind 1 on bodies 1 bodies 1
sketch "スケッチ83" plane through (0, 0, 0) normal (1, 0, 0) x (0, 1, 0)
  line L0 (15, -21) -> (18, -21)
  line L1 (18, -21) -> (18, -2)
  line L2 (18, -2) -> (15, -2)
  line L3 (15, -2) -> (15, -21)
  constraint horizontal L0
  constraint vertical L1
  constraint horizontal L2
  constraint vertical L3
extrude "押し出し65" cut sketch "スケッチ83" against normal blind 2 bodies 1
sketch "スケッチ84" plane through (0, 0, 0) normal (1, 0, 0) x (0, 1, 0)
  line L0 (0, -2) -> (3, -2)
  line L1 (3, -2) -> (3, -21)
  line L2 (3, -21) -> (0, -21)
  line L3 (0, -21) -> (0, -2)
  constraint horizontal L0
  constraint vertical L1
  constraint horizontal L2
  constraint vertical L3
extrude "押し出し66" cut sketch "スケッチ84" against normal blind 3 bodies 1
